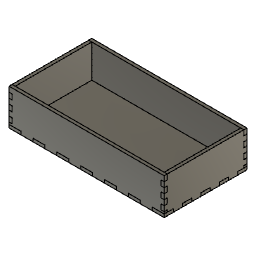
Kassi - Tölvustudd framleiðsla rétt kerf v1 (Autodesk Fusion 360 design; units mm, degrees)
Autodesk Fusion 360 part; units mm, degrees
sketch "Sketch1" plane through (0, 0, 0) normal (0, 0, 1) x (1, 0, 0)
  line L0 (0, 0) -> (-150, 0)
  line L1 (-150, 0) -> (-150, -80)
  line L2 (-150, -80) -> (0, -80)
  line L3 (0, -80) -> (0, 0)
  dimension "d10" = 150
  dimension "d11" = 80
  constraint horizontal L0
  constraint vertical L1
  constraint horizontal L2
  constraint vertical L3
  constraint coincident L0.start L3.end
  measures "d10" distance of L0.start L0.end
  measures "d11" distance of L0.start L2.end
extrude "Extrude1" add sketch "Sketch1" along normal blind 3 makes body 1
sketch "Sketch2" plane through (0, -80, 0) normal (0, -1, 0) x (1, 0, 0)
sketch "Sketch4" plane through (0, 0, 0) normal (0, 1, 0) x (-1, 0, 0)
  line L0 (0, 0) -> (150, 0)
  line L1 (150, 0) -> (150, 3)
  line L2 (150, 3) -> (0, 3)
  line L3 (0, 3) -> (0, 0)
  line L4 (11.5385, 0) -> (23.0769, 0)
  line L5 (23.0769, 0) -> (23.0769, 3)
  line L6 (23.0769, 3) -> (11.5385, 3)
  line L7 (11.5385, 3) -> (11.5385, 0)
  line L8 (34.6154, 3) -> (34.6154, 0)
  line L9 (46.1538, 0) -> (46.1538, 3)
  line L10 (57.6923, 3) -> (57.6923, 0)
  line L11 (69.2308, 0) -> (69.2308, 3)
  line L12 (80.7692, 3) -> (80.7692, 0)
  line L13 (92.3077, 0) -> (92.3077, 3)
  line L14 (103.8462, 3) -> (103.8462, 0)
  line L15 (115.3846, 0) -> (115.3846, 3)
  line L16 (126.9231, 3) -> (126.9231, 0)
  line L17 (138.4615, 0) -> (138.4615, 3)
  line L18 (11.5385, 0) -> (0, 0)
  line L19 (0, 0) -> (0, 3)
  line L20 (0, 3) -> (11.5385, 3)
  line L21 (11.5385, 3) -> (11.5385, 0)
  dimension "d23" = 11.5385
  dimension "d26" = 115.3846
  dimension "d27" = 0
  constraint horizontal L4
  constraint vertical L5
  constraint horizontal L6
  constraint vertical L7
  constraint coincident L2 L5.end
  constraint coincident L0 L4.start
  constraint horizontal L18
  constraint vertical L19
  constraint horizontal L20
  constraint vertical L21
  constraint coincident L2.end L3.start
  measures "d23" distance of L4.start L4.end
extrude "Extrude3" cut sketch "Sketch4" against normal blind 3 contours L0 L2 L4 L5 L6 L7 L21 | L0 L2 L8 L9 | L0 L2 L10 L11 | L0 L2 L12 L13 | L0 L2 L14 L15 | L0 L2 L16 L17 bodies 1
sketch "Sketch5" plane through (0, 0, 0) normal (0, 1, 0) x (1, 0, 0)
  line L0 (0, 0) -> (-150, 0)
  line L1 (-150, 0) -> (-150, -35)
  line L2 (-150, -35) -> (0, -35)
  line L3 (0, -35) -> (0, 0)
  dimension "d31" = 35
  constraint perpendicular L0 L1
  constraint parallel L0 L2
  constraint parallel L1 L3
  constraint horizontal L0
  constraint coincident L0.start L3.end
  measures "d31" distance of L0.start L2.end
extrude "Extrude4" add sketch "Sketch5" against normal blind 3 separate body makes body 2
combine "Combine1" operation cut target body 2 tool bodies 1 keep tools
sketch "Sketch6" plane through (0, 0, 0) normal (1, 0, 0) x (0, 1, 0)
  line L0 (-3, 3) -> (0, 3)
  line L1 (0, 3) -> (0, 35)
  line L2 (0, 35) -> (-3, 35)
  line L3 (-3, 35) -> (-3, 3)
  line L4 (0, 5) -> (-3, 5)
  line L5 (-3, 5) -> (-3, 10)
  line L6 (-3, 10) -> (0, 10)
  line L7 (0, 10) -> (0, 5)
  line L8 (0, 5) -> (-3, 5)
  line L9 (-3, 5) -> (-3, 0)
  line L10 (-3, 0) -> (0, 0)
  line L11 (0, 0) -> (0, 5)
  line L12 (0, 15) -> (-3, 15)
  line L13 (-3, 20) -> (0, 20)
  line L14 (0, 25) -> (-3, 25)
  line L15 (-3, 30) -> (0, 30)
  dimension "d34" = 5
  dimension "d35" = 5
  dimension "d38" = 20
  dimension "d39" = 0
  constraint horizontal L4
  constraint vertical L5
  constraint horizontal L6
  constraint vertical L7
  constraint coincident L3 L5.end
  constraint coincident L1 L4.start
  constraint horizontal L8
  constraint vertical L9
  constraint horizontal L10
  constraint vertical L11
  measures "d34" distance of L4.start L6.end
  measures "d35" distance of L4.start L10.end
extrude "Extrude5" cut sketch "Sketch6" against normal blind 3 contours L1 L3 L4 L5 L6 L7 L8 | L1 L3 L12 L13 | L1 L3 L14 L15 bodies 2
extrude "Extrude6" add 1 faces at (-76.9231, -3, 24.3333) along direction (0, 1, 0) blind 3 from surface at -77 separate body on bodies 2 makes body 3
combine "Combine2" operation cut target body 1 tool bodies 3 keep tools
sketch "Sketch7" plane through (0, 0, 0) normal (1, 0, 0) x (0, 1, 0)
  line L0 (-80, 0) -> (0, 0)
  line L1 (0, 0) -> (0, 35)
  constraint perpendicular L0 L1
  constraint coincident L0.end L1.start
  constraint horizontal L0
sketch "Sketch8" plane through (0, 0, 0) normal (1, 0, 0) x (0, 1, 0)
  line L0 (-80, 0) -> (0, 0)
  line L1 (0, 0) -> (0, 3)
  line L2 (0, 3) -> (-80, 3)
  line L3 (-80, 3) -> (-80, 0)
  line L4 (-71.1111, 0) -> (-62.2222, 0)
  line L5 (-62.2222, 0) -> (-62.2222, 3)
  line L6 (-62.2222, 3) -> (-71.1111, 3)
  line L7 (-71.1111, 3) -> (-71.1111, 0)
  line L8 (-71.1111, 0) -> (-80, 0)
  line L9 (-80, 0) -> (-80, 3)
  line L10 (-80, 3) -> (-71.1111, 3)
  line L11 (-71.1111, 3) -> (-71.1111, 0)
  line L12 (-53.3333, 3) -> (-53.3333, 0)
  line L13 (-44.4444, 0) -> (-44.4444, 3)
  line L14 (-35.5556, 3) -> (-35.5556, 0)
  line L15 (-26.6667, 0) -> (-26.6667, 3)
  line L16 (-17.7778, 3) -> (-17.7778, 0)
  line L17 (-8.8889, 0) -> (-8.8889, 3)
  dimension "d45" = 8.8889
  dimension "d46" = 8.8889
  dimension "d49" = 53.3333
  dimension "d50" = 0
  constraint horizontal L4
  constraint vertical L5
  constraint horizontal L6
  constraint vertical L7
  constraint coincident L0 L4.start
  constraint horizontal L8
  constraint vertical L9
  constraint horizontal L10
  constraint vertical L11
  constraint coincident L2.end L3.start
  measures "d45" distance of L4.start L4.end
  measures "d46" distance of L2.end L6.end
extrude "Extrude7" cut sketch "Sketch8" against normal blind 3 contours L0 L2 L4 L5 L6 L7 L11 | L0 L2 L12 L13 | L0 L2 L14 L15 | L0 L2 L16 L17 bodies 1
sketch "Sketch9" plane through (0, 0, 0) normal (1, 0, 0) x (0, 1, 0)
  line L0 (-80, 0) -> (0, 0)
  line L1 (0, 0) -> (0, 35)
  line L2 (0, 35) -> (-80, 35)
  line L3 (-80, 35) -> (-80, 0)
  constraint perpendicular L0 L1
  constraint parallel L0 L2
  constraint parallel L1 L3
  constraint coincident L0.end L1.start
  constraint horizontal L0
extrude "Extrude8" add sketch "Sketch9" against normal blind 3 separate body makes body 4
combine "Combine3" operation cut target body 4 tool bodies 3 2 1 keep tools
extrude "Extrude9" add 1 faces at (-3, -41.4815, 24.3333) along direction (1, 0, 0) blind 3 from surface at -147 separate body on bodies 4 makes body 5
combine "Combine4" operation cut target body 3 tool bodies 5 keep tools
combine "Combine5" operation cut target body 1 tool bodies 5 keep tools
combine "Combine6" operation cut target body 2 tool bodies 5 keep tools
copy_body "CopyPasteBodies1" bodies 1 2 3 4 5 makes body 6 makes body 7 makes body 8 makes body 9 makes body 10
move_body "Move1" bodies 6 7 8 9 10 to x (1, 0, 0) y (0, 1, 0) z (0, 0, 1) at (0, -130, 0)
move_body "Align1" bodies 8 to x (1, 0, 0) y (0, 0, -1) z (0, 1, 0) at (0, -227.5, -207)
move_body "Move2" bodies 8 to x (1, 0, 0) y (0, 1, 0) z (0, 0, 1) at (0, -40, 0)
move_body "Align2" bodies 9 to x (0, 0, -1) y (0, -1, 0) z (-1, 0, 0) at (-57.5, -340, 3)
move_body "Move3" bodies 9 to x (1, 0, 0) y (0, 1, 0) z (0, 0, 1) at (110, 0, 0)
move_body "Align3" bodies 7 to x (1, 0, 0) y (0, 0, -1) z (0, 1, 0) at (0, -150.5, -130)
move_body "Move4" bodies 7 to x (1, 0, 0) y (0, 1, 0) z (0, 0, 1) at (0, 30, 0)
move_body "Align4" bodies 10 to x (0, 0, 1) y (0, 1, 0) z (-1, 0, 0) at (-129.5, 0, 150)
move_body "Move5" bodies 10 to x (1, 0, 0) y (0, 1, 0) z (0, 0, 1) at (-30, 0, 0)
move_body "Move6" bodies 10 to x (1, 0, 0) y (0, 1, 0) z (0, 0, 1) at (5, 0, 0)
move_body "Move7" bodies 8 to x (1, 0, 0) y (0, 1, 0) z (0, 0, 1) at (0, 20, 0)
move_body "Move8" bodies 9 to x (1, 0, 0) y (0, 1, 0) z (0, 0, 1) at (-10, 0, 0)
move_body "Align5" bodies 7 to x (1, 0, 0) y (0, -1, 0) z (0, 0, -1) at (0, -235, 6)
move_body "Move9" bodies 7 to x (1, 0, 0) y (0, 1, 0) z (0, 0, 1) at (0, 25, 0)
move_body "Align6" bodies 10 to x (-1, 0, 0) y (0, -1, 0) z (0, 0, 1) at (-247, -340, 0)
move_body "Move10" bodies 10 to x (1, 0, 0) y (0, 1, 0) z (0, 0, 1) at (-100, 0, 0)
sketch "Sketch10" plane through (0, 0, 3) normal (0, 0, 1) x (-1, 0, 0)
  line L0 (150, 130) -> (150, 138.8889)
  line L1 (150, 138.8889) -> (147, 138.8889)
  line L2 (147, 138.8889) -> (147, 147.7778)
  line L3 (147, 147.7778) -> (150, 147.7778)
  line L4 (150, 147.7778) -> (150, 156.6667)
  line L5 (150, 156.6667) -> (147, 156.6667)
  line L6 (147, 156.6667) -> (147, 165.5556)
  line L7 (147, 165.5556) -> (150, 165.5556)
  line L8 (150, 165.5556) -> (150, 174.4444)
  line L9 (150, 174.4444) -> (147, 174.4444)
  line L10 (147, 174.4444) -> (147, 183.3333)
  line L11 (147, 183.3333) -> (150, 183.3333)
  line L12 (150, 183.3333) -> (150, 192.2222)
  line L13 (150, 192.2222) -> (147, 192.2222)
  line L14 (147, 192.2222) -> (147, 201.1111)
  line L15 (147, 201.1111) -> (150, 201.1111)
  line L16 (150, 201.1111) -> (150, 210)
  line L17 (150, 210) -> (138.4615, 210)
  line L18 (138.4615, 210) -> (138.4615, 207)
  line L19 (138.4615, 207) -> (126.9231, 207)
  line L20 (126.9231, 207) -> (126.9231, 210)
  line L21 (126.9231, 210) -> (115.3846, 210)
  line L22 (115.3846, 210) -> (115.3846, 207)
  line L23 (115.3846, 207) -> (103.8462, 207)
  line L24 (103.8462, 207) -> (103.8462, 210)
  line L25 (103.8462, 210) -> (92.3077, 210)
  line L26 (92.3077, 210) -> (92.3077, 207)
  line L27 (92.3077, 207) -> (80.7692, 207)
  line L28 (80.7692, 207) -> (80.7692, 210)
  line L29 (80.7692, 210) -> (69.2308, 210)
  line L30 (69.2308, 210) -> (69.2308, 207)
  line L31 (69.2308, 207) -> (57.6923, 207)
  line L32 (57.6923, 207) -> (57.6923, 210)
  line L33 (57.6923, 210) -> (46.1538, 210)
  line L34 (46.1538, 210) -> (46.1538, 207)
  line L35 (46.1538, 207) -> (34.6154, 207)
  line L36 (34.6154, 207) -> (34.6154, 210)
  line L37 (34.6154, 210) -> (23.0769, 210)
  line L38 (23.0769, 210) -> (23.0769, 207)
  line L39 (23.0769, 207) -> (11.5385, 207)
  line L40 (11.5385, 207) -> (11.5385, 210)
  line L41 (11.5385, 210) -> (0, 210)
  line L42 (0, 210) -> (0, 201.1111)
  line L43 (0, 201.1111) -> (3, 201.1111)
  line L44 (3, 201.1111) -> (3, 192.2222)
  line L45 (3, 192.2222) -> (0, 192.2222)
  line L46 (0, 192.2222) -> (0, 183.3333)
  line L47 (0, 183.3333) -> (3, 183.3333)
  line L48 (3, 183.3333) -> (3, 174.4444)
  line L49 (3, 174.4444) -> (0, 174.4444)
  line L50 (0, 174.4444) -> (0, 165.5556)
  line L51 (0, 165.5556) -> (3, 165.5556)
  line L52 (3, 165.5556) -> (3, 156.6667)
  line L53 (3, 156.6667) -> (0, 156.6667)
  line L54 (0, 156.6667) -> (0, 147.7778)
  line L55 (0, 147.7778) -> (3, 147.7778)
  line L56 (3, 147.7778) -> (3, 138.8889)
  line L57 (3, 138.8889) -> (0, 138.8889)
  line L58 (0, 138.8889) -> (0, 130)
  line L59 (0, 130) -> (11.5385, 130)
  line L60 (11.5385, 130) -> (11.5385, 133)
  line L61 (11.5385, 133) -> (23.0769, 133)
  line L62 (23.0769, 133) -> (23.0769, 130)
  line L63 (23.0769, 130) -> (34.6154, 130)
  line L64 (34.6154, 130) -> (34.6154, 133)
  line L65 (34.6154, 133) -> (46.1538, 133)
  line L66 (46.1538, 133) -> (46.1538, 130)
  line L67 (46.1538, 130) -> (57.6923, 130)
  line L68 (57.6923, 130) -> (57.6923, 133)
  line L69 (57.6923, 133) -> (69.2308, 133)
  line L70 (69.2308, 133) -> (69.2308, 130)
  line L71 (69.2308, 130) -> (80.7692, 130)
  line L72 (80.7692, 130) -> (80.7692, 133)
  line L73 (80.7692, 133) -> (92.3077, 133)
  line L74 (92.3077, 133) -> (92.3077, 130)
  line L75 (92.3077, 130) -> (103.8462, 130)
  line L76 (103.8462, 130) -> (103.8462, 133)
  line L77 (103.8462, 133) -> (115.3846, 133)
  line L78 (115.3846, 133) -> (115.3846, 130)
  line L79 (115.3846, 130) -> (126.9231, 130)
  line L80 (126.9231, 130) -> (126.9231, 133)
  line L81 (126.9231, 133) -> (138.4615, 133)
  line L82 (138.4615, 133) -> (138.4615, 130)
  line L83 (138.4615, 130) -> (150, 130)
  line L84 (147, 165.5556) -> (147, 156.6667)
  line L85 (147, 183.3333) -> (147, 174.4444)
  line L86 (147, 201.1111) -> (147, 192.2222)
  line L87 (147, 147.7778) -> (147, 138.8889)
  line L88 (147, 138.8889) -> (150, 138.8889)
  line L89 (150, 147.7778) -> (147, 147.7778)
  line L90 (147, 156.6667) -> (150, 156.6667)
  line L91 (150, 165.5556) -> (147, 165.5556)
  line L92 (147, 174.4444) -> (150, 174.4444)
  line L93 (150, 183.3333) -> (147, 183.3333)
  line L94 (147, 192.2222) -> (150, 192.2222)
  line L95 (150, 201.1111) -> (147, 201.1111)
  line L96 (150, 201.1111) -> (150, 210)
  line L97 (150, 183.3333) -> (150, 192.2222)
  line L98 (150, 165.5556) -> (150, 174.4444)
  line L99 (150, 147.7778) -> (150, 156.6667)
  line L100 (150, 130) -> (150, 138.8889)
  line L101 (3, 183.3333) -> (0, 183.3333)
  line L102 (0, 174.4444) -> (3, 174.4444)
  line L103 (3, 174.4444) -> (3, 183.3333)
  line L104 (3, 165.5556) -> (0, 165.5556)
  line L105 (0, 156.6667) -> (3, 156.6667)
  line L106 (3, 156.6667) -> (3, 165.5556)
  line L107 (0, 192.2222) -> (3, 192.2222)
  line L108 (3, 201.1111) -> (0, 201.1111)
  line L109 (3, 192.2222) -> (3, 201.1111)
  line L110 (3, 147.7778) -> (0, 147.7778)
  line L111 (0, 138.8889) -> (3, 138.8889)
  line L112 (3, 138.8889) -> (3, 147.7778)
  line L113 (0, 138.8889) -> (0, 130)
  line L114 (0, 210) -> (0, 201.1111)
  line L115 (0, 156.6667) -> (0, 147.7778)
  line L116 (0, 192.2222) -> (0, 183.3333)
  line L117 (0, 174.4444) -> (0, 165.5556)
  line L118 (138.4615, 130) -> (150, 130)
  line L119 (138.4615, 130) -> (138.4615, 133)
  line L120 (138.4615, 133) -> (126.9231, 133)
  line L121 (126.9231, 133) -> (126.9231, 130)
  line L122 (115.3846, 130) -> (126.9231, 130)
  line L123 (115.3846, 130) -> (115.3846, 133)
  line L124 (115.3846, 133) -> (103.8462, 133)
  line L125 (103.8462, 133) -> (103.8462, 130)
  line L126 (92.3077, 130) -> (103.8462, 130)
  line L127 (92.3077, 130) -> (92.3077, 133)
  line L128 (92.3077, 133) -> (80.7692, 133)
  line L129 (80.7692, 133) -> (80.7692, 130)
  line L130 (69.2308, 130) -> (80.7692, 130)
  line L131 (69.2308, 130) -> (69.2308, 133)
  line L132 (69.2308, 133) -> (57.6923, 133)
  line L133 (57.6923, 133) -> (57.6923, 130)
  line L134 (46.1538, 130) -> (57.6923, 130)
  line L135 (46.1538, 130) -> (46.1538, 133)
  line L136 (46.1538, 133) -> (34.6154, 133)
  line L137 (34.6154, 133) -> (34.6154, 130)
  line L138 (23.0769, 130) -> (34.6154, 130)
  line L139 (23.0769, 130) -> (23.0769, 133)
  line L140 (23.0769, 133) -> (11.5385, 133)
  line L141 (11.5385, 133) -> (11.5385, 130)
  line L142 (0, 130) -> (11.5385, 130)
  line L143 (11.5385, 210) -> (0, 210)
  line L144 (11.5385, 210) -> (11.5385, 207)
  line L145 (11.5385, 207) -> (23.0769, 207)
  line L146 (23.0769, 207) -> (23.0769, 210)
  line L147 (34.6154, 210) -> (23.0769, 210)
  line L148 (34.6154, 210) -> (34.6154, 207)
  line L149 (34.6154, 207) -> (46.1538, 207)
  line L150 (46.1538, 207) -> (46.1538, 210)
  line L151 (57.6923, 210) -> (46.1538, 210)
  line L152 (57.6923, 210) -> (57.6923, 207)
  line L153 (57.6923, 207) -> (69.2308, 207)
  line L154 (69.2308, 207) -> (69.2308, 210)
  line L155 (80.7692, 210) -> (69.2308, 210)
  line L156 (80.7692, 210) -> (80.7692, 207)
  line L157 (80.7692, 207) -> (92.3077, 207)
  line L158 (92.3077, 207) -> (92.3077, 210)
  line L159 (103.8462, 210) -> (92.3077, 210)
  line L160 (103.8462, 210) -> (103.8462, 207)
  line L161 (103.8462, 207) -> (115.3846, 207)
  line L162 (115.3846, 207) -> (115.3846, 210)
  line L163 (126.9231, 210) -> (115.3846, 210)
  line L164 (126.9231, 210) -> (126.9231, 207)
  line L165 (126.9231, 207) -> (138.4615, 207)
  line L166 (138.4615, 207) -> (138.4615, 210)
  line L167 (150, 210) -> (138.4615, 210)
  line L168 (147, 109.5) -> (147, 104.5)
  line L169 (147, 99.5) -> (147, 94.5)
  line L170 (147, 119.5) -> (147, 114.5)
  line L171 (150, 119.5) -> (147, 119.5)
  line L172 (147, 114.5) -> (150, 114.5)
  line L173 (150, 109.5) -> (147, 109.5)
  line L174 (147, 104.5) -> (150, 104.5)
  line L175 (150, 99.5) -> (147, 99.5)
  line L176 (147, 94.5) -> (150, 94.5)
  line L177 (150, 114.5) -> (150, 109.5)
  line L178 (150, 104.5) -> (150, 99.5)
  line L179 (150, 94.5) -> (150, 92.5)
  line L180 (150, 92.5) -> (138.4615, 92.5)
  line L181 (138.4615, 92.5) -> (138.4615, 89.5)
  line L182 (138.4615, 89.5) -> (126.9231, 89.5)
  line L183 (126.9231, 89.5) -> (126.9231, 92.5)
  line L184 (126.9231, 92.5) -> (115.3846, 92.5)
  line L185 (115.3846, 92.5) -> (115.3846, 89.5)
  line L186 (115.3846, 89.5) -> (103.8462, 89.5)
  line L187 (103.8462, 89.5) -> (103.8462, 92.5)
  line L188 (103.8462, 92.5) -> (92.3077, 92.5)
  line L189 (92.3077, 92.5) -> (92.3077, 89.5)
  line L190 (92.3077, 89.5) -> (80.7692, 89.5)
  line L191 (80.7692, 89.5) -> (80.7692, 92.5)
  line L192 (80.7692, 92.5) -> (69.2308, 92.5)
  line L193 (69.2308, 92.5) -> (69.2308, 89.5)
  line L194 (69.2308, 89.5) -> (57.6923, 89.5)
  line L195 (57.6923, 89.5) -> (57.6923, 92.5)
  line L196 (57.6923, 92.5) -> (46.1538, 92.5)
  line L197 (46.1538, 92.5) -> (46.1538, 89.5)
  line L198 (46.1538, 89.5) -> (34.6154, 89.5)
  line L199 (34.6154, 89.5) -> (34.6154, 92.5)
  line L200 (34.6154, 92.5) -> (23.0769, 92.5)
  line L201 (23.0769, 92.5) -> (23.0769, 89.5)
  line L202 (23.0769, 89.5) -> (11.5385, 89.5)
  line L203 (11.5385, 89.5) -> (11.5385, 92.5)
  line L204 (11.5385, 92.5) -> (0, 92.5)
  line L205 (0, 92.5) -> (0, 94.5)
  line L206 (0, 94.5) -> (3, 94.5)
  line L207 (3, 94.5) -> (3, 99.5)
  line L208 (3, 99.5) -> (0, 99.5)
  line L209 (0, 99.5) -> (0, 104.5)
  line L210 (0, 104.5) -> (3, 104.5)
  line L211 (3, 104.5) -> (3, 109.5)
  line L212 (3, 109.5) -> (0, 109.5)
  line L213 (0, 109.5) -> (0, 114.5)
  line L214 (0, 114.5) -> (3, 114.5)
  line L215 (3, 114.5) -> (3, 119.5)
  line L216 (3, 119.5) -> (0, 119.5)
  line L217 (0, 119.5) -> (0, 124.5)
  line L218 (0, 124.5) -> (150, 124.5)
  line L219 (150, 124.5) -> (150, 119.5)
  line L220 (189.5, 201.1111) -> (189.5, 207)
  line L221 (192.5, 201.1111) -> (189.5, 201.1111)
  line L222 (192.5, 192.2222) -> (192.5, 201.1111)
  line L223 (189.5, 192.2222) -> (192.5, 192.2222)
  line L224 (189.5, 183.3333) -> (189.5, 192.2222)
  line L225 (192.5, 183.3333) -> (189.5, 183.3333)
  line L226 (192.5, 174.4444) -> (192.5, 183.3333)
  line L227 (189.5, 174.4444) -> (192.5, 174.4444)
  line L228 (189.5, 165.5556) -> (189.5, 174.4444)
  line L229 (192.5, 165.5556) -> (189.5, 165.5556)
  line L230 (192.5, 156.6667) -> (192.5, 165.5556)
  line L231 (189.5, 156.6667) -> (192.5, 156.6667)
  line L232 (189.5, 147.7778) -> (189.5, 156.6667)
  line L233 (192.5, 147.7778) -> (189.5, 147.7778)
  line L234 (192.5, 138.8889) -> (192.5, 147.7778)
  line L235 (189.5, 138.8889) -> (192.5, 138.8889)
  line L236 (189.5, 133) -> (189.5, 138.8889)
  line L237 (187.5, 133) -> (189.5, 133)
  line L238 (187.5, 130) -> (187.5, 133)
  line L239 (182.5, 130) -> (187.5, 130)
  line L240 (182.5, 133) -> (182.5, 130)
  line L241 (177.5, 133) -> (182.5, 133)
  line L242 (177.5, 130) -> (177.5, 133)
  line L243 (172.5, 130) -> (177.5, 130)
  line L244 (172.5, 133) -> (172.5, 130)
  line L245 (167.5, 133) -> (172.5, 133)
  line L246 (167.5, 130) -> (167.5, 133)
  line L247 (162.5, 130) -> (167.5, 130)
  line L248 (162.5, 133) -> (162.5, 130)
  line L249 (157.5, 133) -> (162.5, 133)
  line L250 (157.5, 207) -> (157.5, 133)
  line L251 (162.5, 207) -> (157.5, 207)
  line L252 (162.5, 210) -> (162.5, 207)
  line L253 (167.5, 210) -> (162.5, 210)
  line L254 (167.5, 207) -> (167.5, 210)
  line L255 (172.5, 207) -> (167.5, 207)
  line L256 (172.5, 210) -> (172.5, 207)
  line L257 (177.5, 210) -> (172.5, 210)
  line L258 (177.5, 207) -> (177.5, 210)
  line L259 (182.5, 207) -> (177.5, 207)
  line L260 (182.5, 210) -> (182.5, 207)
  line L261 (187.5, 210) -> (182.5, 210)
  line L262 (187.5, 207) -> (187.5, 210)
  line L263 (189.5, 207) -> (187.5, 207)
  line L264 (147, 232.5) -> (147, 227.5)
  line L265 (147, 222.5) -> (147, 217.5)
  line L266 (147, 242.5) -> (147, 237.5)
  line L267 (150, 242.5) -> (147, 242.5)
  line L268 (147, 237.5) -> (150, 237.5)
  line L269 (150, 232.5) -> (147, 232.5)
  line L270 (147, 227.5) -> (150, 227.5)
  line L271 (150, 222.5) -> (147, 222.5)
  line L272 (147, 217.5) -> (150, 217.5)
  line L273 (150, 217.5) -> (150, 212.5)
  line L274 (150, 227.5) -> (150, 222.5)
  line L275 (150, 237.5) -> (150, 232.5)
  line L276 (150, 244.5) -> (150, 242.5)
  line L277 (150, 212.5) -> (0, 212.5)
  line L278 (0, 212.5) -> (0, 217.5)
  line L279 (0, 217.5) -> (3, 217.5)
  line L280 (3, 217.5) -> (3, 222.5)
  line L281 (3, 222.5) -> (0, 222.5)
  line L282 (0, 222.5) -> (0, 227.5)
  line L283 (0, 227.5) -> (3, 227.5)
  line L284 (3, 227.5) -> (3, 232.5)
  line L285 (3, 232.5) -> (0, 232.5)
  line L286 (0, 232.5) -> (0, 237.5)
  line L287 (0, 237.5) -> (3, 237.5)
  line L288 (3, 237.5) -> (3, 242.5)
  line L289 (3, 242.5) -> (0, 242.5)
  line L290 (0, 242.5) -> (0, 244.5)
  line L291 (0, 244.5) -> (11.5385, 244.5)
  line L292 (11.5385, 244.5) -> (11.5385, 247.5)
  line L293 (11.5385, 247.5) -> (23.0769, 247.5)
  line L294 (23.0769, 247.5) -> (23.0769, 244.5)
  line L295 (23.0769, 244.5) -> (34.6154, 244.5)
  line L296 (34.6154, 244.5) -> (34.6154, 247.5)
  line L297 (34.6154, 247.5) -> (46.1538, 247.5)
  line L298 (46.1538, 247.5) -> (46.1538, 244.5)
  line L299 (46.1538, 244.5) -> (57.6923, 244.5)
  line L300 (57.6923, 244.5) -> (57.6923, 247.5)
  line L301 (57.6923, 247.5) -> (69.2308, 247.5)
  line L302 (69.2308, 247.5) -> (69.2308, 244.5)
  line L303 (69.2308, 244.5) -> (80.7692, 244.5)
  line L304 (80.7692, 244.5) -> (80.7692, 247.5)
  line L305 (80.7692, 247.5) -> (92.3077, 247.5)
  line L306 (92.3077, 247.5) -> (92.3077, 244.5)
  line L307 (92.3077, 244.5) -> (103.8462, 244.5)
  line L308 (103.8462, 244.5) -> (103.8462, 247.5)
  line L309 (103.8462, 247.5) -> (115.3846, 247.5)
  line L310 (115.3846, 247.5) -> (115.3846, 244.5)
  line L311 (115.3846, 244.5) -> (126.9231, 244.5)
  line L312 (126.9231, 244.5) -> (126.9231, 247.5)
  line L313 (126.9231, 247.5) -> (138.4615, 247.5)
  line L314 (138.4615, 247.5) -> (138.4615, 244.5)
  line L315 (138.4615, 244.5) -> (150, 244.5)
  line L316 (-39.5, 201.1111) -> (-39.5, 207)
  line L317 (-39.5, 183.3333) -> (-39.5, 192.2222)
  line L318 (-39.5, 165.5556) -> (-39.5, 174.4444)
  line L319 (-39.5, 147.7778) -> (-39.5, 156.6667)
  line L320 (-39.5, 133) -> (-39.5, 138.8889)
  line L321 (-39.5, 156.6667) -> (-42.5, 156.6667)
  line L322 (-42.5, 165.5556) -> (-39.5, 165.5556)
  line L323 (-39.5, 174.4444) -> (-42.5, 174.4444)
  line L324 (-42.5, 183.3333) -> (-39.5, 183.3333)
  line L325 (-42.5, 147.7778) -> (-39.5, 147.7778)
  line L326 (-39.5, 138.8889) -> (-42.5, 138.8889)
  line L327 (-39.5, 192.2222) -> (-42.5, 192.2222)
  line L328 (-42.5, 201.1111) -> (-39.5, 201.1111)
  line L329 (-42.5, 138.8889) -> (-42.5, 147.7778)
  line L330 (-42.5, 156.6667) -> (-42.5, 165.5556)
  line L331 (-42.5, 174.4444) -> (-42.5, 183.3333)
  line L332 (-12.5, 207) -> (-7.5, 207)
  line L333 (-22.5, 207) -> (-17.5, 207)
  line L334 (-32.5, 207) -> (-27.5, 207)
  line L335 (-32.5, 210) -> (-32.5, 207)
  line L336 (-37.5, 207) -> (-37.5, 210)
  line L337 (-22.5, 210) -> (-22.5, 207)
  line L338 (-27.5, 207) -> (-27.5, 210)
  line L339 (-12.5, 210) -> (-12.5, 207)
  line L340 (-17.5, 207) -> (-17.5, 210)
  line L341 (-39.5, 207) -> (-37.5, 207)
  line L342 (-7.5, 207) -> (-7.5, 133)
  line L343 (-17.5, 210) -> (-12.5, 210)
  line L344 (-27.5, 210) -> (-22.5, 210)
  line L345 (-37.5, 210) -> (-32.5, 210)
  line L346 (-37.5, 133) -> (-39.5, 133)
  line L347 (-27.5, 133) -> (-32.5, 133)
  line L348 (-17.5, 133) -> (-22.5, 133)
  line L349 (-32.5, 133) -> (-32.5, 130)
  line L350 (-27.5, 130) -> (-27.5, 133)
  line L351 (-22.5, 133) -> (-22.5, 130)
  line L352 (-17.5, 130) -> (-17.5, 133)
  line L353 (-12.5, 133) -> (-12.5, 130)
  line L354 (-37.5, 130) -> (-37.5, 133)
  line L355 (-7.5, 133) -> (-12.5, 133)
  line L356 (-12.5, 130) -> (-17.5, 130)
  line L357 (-22.5, 130) -> (-27.5, 130)
  line L358 (-32.5, 130) -> (-37.5, 130)
  line L359 (-42.5, 192.2222) -> (-42.5, 201.1111)
hidden bodies 6 7 8 9 10
equation "lengd = 150 mm"
equation "breidd = 80 mm"
equation "hæð = 35 mm"
equation "lputti = 6"
equation "bputti = 4"
equation "hputti = 3"
equation "lputtiw = lengd / ( ( lputti * 2 ) + 1 )"
equation "bputtiw = breidd / ( ( bputti * 2 ) + 1 )"
equation "hputtiw = hæð / ( ( hputti * 2 ) + 1 )"
equation "d10 = lengd"
equation "d11 = breidd"
equation "þykkt = 3 mm"
equation "d13 = þykkt"
equation "d23 = lputtiw"
equation "d24 = lputti"
equation "d26 = lengd - lputtiw * 3"
equation "d29 = -þykkt"
equation "d31 = hæð"
equation "d32 = -þykkt"
equation "d34 = hputtiw"
equation "d35 = hputtiw"
equation "d38 = hæð - hputtiw * 3"
equation "d40 = -þykkt"
equation "d43 = -þykkt"
equation "d45 = bputtiw"
equation "d46 = bputtiw"
equation "d47 = bputti"
equation "d49 = breidd - bputtiw * 3"
equation "d51 = -þykkt"
equation "d53 = -þykkt"
equation "d56 = -þykkt"
